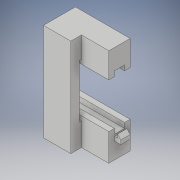
# Autodesk Inventor part: EngineClipTestBlock
Saved by Autodesk Inventor 2018 (Build 220112000, 112)
## iProperties
Created: 2019-08-29
Part Number: EngineClipTestBlock
Material: Generic
Document SubType Name: Modeling
Designer: 871357
Density: 1 g/cm^3
Appearance: Default
Author: 871357
Autodesk Inventor part; units mm, degrees
ref_plane "YZ Plane" through (0, 0, 0) normal (1, 0, 0) x (0, 1, 0)
ref_plane "XZ Plane" through (0, 0, 0) normal (0, 1, 0) x (-1, 0, 0)
sketch "Sketch1" plane through (0, 0, 0) normal (1, 0, 0) x (0, 1, 0)
  line L0 (0, 0) -> (228.6, 0)
  line L1 (228.6, 0) -> (228.6, -424.18)
  line L2 (228.6, -424.18) -> (0, -424.18)
  line L3 (0, -424.18) -> (0, 0)
  point P0 (0, 0)
  dimension "d0" = 424.18
  dimension "d1" = 228.6
  constraints: 8 end point, 2 parallel, 1 coincident, 1 horizontal, 1 perpendicular
  measures "d0" distance of L0.end L1.end
  measures "d1" distance of L0.start L0.end
extrude "Extrusion1" add sketch "Sketch1" along normal blind 165.1
sketch "Sketch2" plane through (165.1, 0, 0) normal (1, 0, 0) x (0, 0, -1)
  line L0 (0, 0) -> (424.18, 0) construction
  line L1 (12.7, 0) -> (411.48, 0)
  line L2 (411.48, 0) -> (411.48, 165.1)
  line L3 (411.48, 165.1) -> (12.7, 165.1)
  line L4 (12.7, 165.1) -> (12.7, 0)
  line L5 (0, 228.6) -> (0, 0) construction
  line L6 (424.18, 0) -> (424.18, 228.6) construction
  dimension "d4" = 398.78
  dimension "d5" = 165.1
  dimension "d6" = 12.7
  dimension "d7" = 12.7
  constraints: 8 end point, 2 parallel, 1 horizontal, 1 perpendicular, 1 point on line
  measures "d4" distance of L3.end L2.end
  measures "d5" distance of L2.end L1.end
  measures "d6" distance between parallel lines of L5 L4
  measures "d7" distance between parallel lines of L6 L2
extrude "Extrusion2" cut sketch "Sketch2" against normal blind 148.59
sketch "Sketch3" plane through (0, 0, 0) normal (0, 0, 1) x (1, 0, 0)
  line L0 (165.1, 228.6) -> (165.1, 0) projected
  line L1 (165.1, 89.535) -> (82.55, 89.535)
  line L2 (69.215, 89.535) -> (69.215, 62.865) construction
  line L3 (82.55, 62.865) -> (165.1, 62.865)
  line L4 (165.1, 62.865) -> (165.1, 89.535)
  line L5 (0, 0) -> (165.1, 0) projected
  arc A0 (82.55, 89.535) -> (82.55, 62.865) centre (82.55, 76.2) ccw
  dimension "d10" = 95.885
  dimension "d11" = 26.67
  dimension "d12" = 62.865
  constraints: 8 end point, 3 tangent, 2 parallel, 2 point on circle, 1 centre point, 1 horizontal, 1 perpendicular, 1 point on line
  measures "d10" distance between parallel lines of L0 L2
  measures "d11" distance of L2.start L2.end
  measures "d12" distance between parallel lines of L5 L3
extrude "Extrusion3" cut sketch "Sketch3" against normal blind 457.2
sketch "Sketch4" plane through (0, 228.6, 0) normal (0, 1, 0) x (1, 0, 0)
  line L0 (165.1, 12.7) -> (165.1, 411.48) construction
  line L1 (165.1, 12.7) -> (16.51, 12.7) construction
  line L2 (16.51, 12.7) -> (16.51, 411.48) construction
  line L3 (165.1, 411.48) -> (16.51, 411.48) construction
  line L4 (0, 424.18) -> (165.1, 424.18) construction
  line L5 (0, 424.18) -> (165.1, 424.18) construction
  circle A0 centre (82.55, 353.06) radius 43.815
  line L6 (0, 0) -> (0, 424.18) construction
  circle A1 centre (82.55, 259.08) radius 43.815
  line L7 (0, 212.09) -> (165.1, 212.09) construction
  line L8 (165.1, 424.18) -> (165.1, 0) construction
  circle A2 centre (82.55, 71.12) radius 43.815
  circle A3 centre (82.55, 165.1) radius 43.815
  dimension "d15" = 87.63
  dimension "d16" = 82.55
  dimension "d17" = 58.42
  dimension "d18" = 87.63
  dimension "d19" = 93.98
  dimension "d20" = 82.55
  constraints: 4 centre point, 4 end point, 2 midpoint, 2 symmetric about line, 1 collinear, 2 other
  measures "d15" diameter of A0
  measures "d16" distance from line of L6 A0.centre
  measures "d17" distance from line of L3 A0.centre
  measures "d18" diameter of A1
  measures "d19" distance of A0.centre A1.centre
  measures "d20" distance from line of L0 A1.centre
extrude "Extrusion4" cut sketch "Sketch4" against normal blind 76.2
sketch "Sketch5" plane through (0, 228.6, 0) normal (0, 1, 0) x (1, 0, 0)
  circle A0 centre (82.55, 165.1) radius 43.815 projected
  circle A1 centre (82.55, 353.06) radius 43.815 projected
  circle A2 centre (82.55, 259.08) radius 43.815 projected
  circle A3 centre (82.55, 71.12) radius 43.815 projected
  line L0 (0, 0) -> (0, 424.18) projected
  line L1 (0, 0) -> (165.1, 0) projected
  line L2 (165.1, 424.18) -> (165.1, 0) projected
  line L3 (0, 424.18) -> (165.1, 424.18) projected
  point P0 (0, 0)
extrude "Extrusion5" add sketch "Sketch5" along normal blind 53.34
sketch "Sketch7" plane through (0, 0, 0) normal (-1, 0, 0) x (0, 0, 1)
  line L0 (0, 0) -> (0, 281.94) projected
  line L1 (-424.18, 281.94) -> (0, 281.94) projected
  line L2 (-424.18, 281.94) -> (-424.18, 0) projected
  line L3 (-424.18, 0) -> (0, 0) projected
  point P0 (0, 0)
extrude "Extrusion6" add sketch "Sketch7" along normal blind 19.05
sketch "Sketch8" plane through (16.51, 0, 0) normal (1, 0, 0) x (0, 0, -1)
  line L0 (411.48, 0) -> (12.7, 0) projected
  line L1 (411.48, 165.1) -> (411.48, 0) projected
  line L2 (12.7, 165.1) -> (411.48, 165.1) projected
  line L3 (12.7, 0) -> (12.7, 165.1) projected
  point P0 (0, 0)
extrude "Extrusion7" cut sketch "Sketch8" against normal blind 19.05
sketch "Sketch12" plane through (165.1, 0, 0) normal (1, 0, 0) x (0, 0, -1)
  line L0 (0, 89.535) -> (12.7, 89.535) construction
  line L1 (3.302, 89.535) -> (9.398, 89.535)
  line L2 (9.398, 89.535) -> (9.398, 92.583)
  line L3 (9.398, 92.583) -> (3.302, 92.583)
  line L4 (3.302, 92.583) -> (3.302, 89.535)
  line L5 (0, 89.535) -> (0, 281.94) construction
  line L6 (12.7, 89.535) -> (12.7, 62.865) construction
  line L7 (0, 89.535) -> (12.7, 89.535) construction
  line L8 (0, 62.865) -> (0, 89.535) construction
  line L9 (0, 62.865) -> (12.7, 62.865) construction
  line L10 (0, 62.865) -> (0, 89.535) construction
  line L11 (0, 76.2) -> (12.7, 76.2) construction
  line L12 (3.302, 62.865) -> (9.398, 62.865)
  line L13 (9.398, 62.865) -> (9.398, 59.817)
  line L14 (9.398, 59.817) -> (3.302, 59.817)
  line L15 (3.302, 59.817) -> (3.302, 62.865)
  point P0 (0, 0)
  dimension "d44" = 6.096
  dimension "d45" = 3.048
  dimension "d46" = 3.302
  constraints: 18 end point, 4 symmetric about line, 2 midpoint, 2 parallel, 1 horizontal, 1 perpendicular, 1 point on line
  measures "d44" distance of L3.end L2.end
  measures "d45" distance of L2.end L1.end
  measures "d46" distance between parallel lines of L5 L4
extrude "Extrusion11" cut sketch "Sketch12" against normal blind 82.55
sketch "Sketch13" plane through (-19.05, 0, 0) normal (0, -1, 0) x (1, 0, 0)
  line L0 (16.51, -12.7) -> (184.15, -12.7) projected
  line L1 (184.15, 0) -> (184.15, -12.7) projected
  line L2 (0, 0) -> (184.15, 0) projected
  line L3 (0, -424.18) -> (0, 0) projected
  line L4 (184.15, -424.18) -> (0, -424.18) projected
  line L5 (184.15, -411.48) -> (184.15, -424.18) projected
  line L6 (184.15, -411.48) -> (16.51, -411.48) projected
  line L7 (16.51, -411.48) -> (16.51, -12.7) projected
  point P0 (19.05, 0)
extrude "Extrusion12" add sketch "Sketch13" along normal blind 5.08
ref_plane "Work Plane1" through (82.55, 89.535, -212.09) normal (0, 0, 1) x (1, 0, 0)
mirror "Mirror1" about plane through (82.55, 89.535, -212.09) normal (0, 0, 1) of "Extrusion11"
sketch "Sketch15" plane through (165.1, 0, 0) normal (1, 0, 0) x (0, 0, -1)
  line L0 (3.302, 59.817) -> (8.89, 59.817)
  line L1 (8.89, 59.817) -> (8.89, 57.912)
  line L2 (8.89, 57.912) -> (3.302, 57.912)
  line L3 (3.302, 57.912) -> (3.302, 59.817)
  line L4 (9.398, 59.817) -> (3.302, 59.817) projected
  point P0 (0, 0)
  dimension "d55" = 5.588
  dimension "d56" = 1.905
  constraints: 8 end point, 2 parallel, 1 horizontal, 1 perpendicular
  measures "d55" distance of L1.end L2.end
  measures "d56" distance of L0.end L1.end
extrude "Extrusion14" add sketch "Sketch15" along normal blind 3.81
sketch "Sketch17" plane through (165.1, 57.912, -3.302) normal (0, 0, 1) x (1, 0, 0)
  line L0 (0, 1.905) -> (3.81, 1.905) projected
  line L1 (3.81, 1.905) -> (0, 1.905)
  line L2 (0, 1.905) -> (0, 0.889)
  line L3 (0, 0.889) -> (3.81, 0.889)
  line L4 (3.81, 0.889) -> (3.81, 1.905)
  point P0 (-165.1, -57.912)
  dimension "d60" = 3.81
  dimension "d61" = 1.016
  constraints: 8 end point, 2 parallel, 1 horizontal, 1 perpendicular
  measures "d60" distance of L3.end L2.end
  measures "d61" distance of L2.end L1.end
extrude "Extrusion15" cut sketch "Sketch17" against normal blind 25.4
sketch "Sketch18" plane through (165.1, 57.912, -3.302) normal (0, 0, 1) x (1, 0, 0)
  line L0 (0, 1.905) -> (-82.55, 1.905) construction
  line L1 (3.81, 0) -> (3.81, 0.889) projected
  line L2 (1.905, 2.9464) -> (3.81, 0.889)
  line L3 (3.81, 0.889) -> (1.905, 0.889)
  line L4 (1.905, 0.889) -> (1.905, 2.9464)
  line L5 (0, 4.953) -> (0, -62.992) projected
  point P0 (-165.1, -57.912)
  dimension "d64" = 1.905
  dimension "d65" = 2.0574
  constraints: 6 end point, 2 perpendicular
  measures "d64" distance between parallel lines of L4 L5
  measures "d65" distance of L3.end L2.start
extrude "Extrusion16" add sketch "Sketch18" against normal blind 5.588
sketch "Sketch19" plane through (165.1, 57.912, -8.89) normal (0, -1, 0) x (1, 0, 0)
  line L0 (0, 0) -> (0, 5.588) projected
  line L1 (0, 0) -> (3.81, 0) projected
  line L2 (3.81, 5.588) -> (3.81, 0) projected
  line L3 (0, 5.588) -> (3.81, 5.588) projected
  point P0 (-165.1, 8.89)
extrude "Extrusion17" add sketch "Sketch19" along normal blind 1.524
mirror "Mirror2" about plane through (82.55, 89.535, -212.09) normal (0, 0, 1) of "Extrusion14", "Extrusion15", "Extrusion16", "Extrusion17"
sketch "Sketch21" plane through (82.55, 89.535, 0) normal (0, 0, 1) x (1, 0, 0)
  line L0 (49.9587, -43.0228) -> (93.9109, -43.0228)
  line L1 (93.9109, -43.0228) -> (93.9109, 15.0648)
  line L2 (93.9109, 15.0648) -> (49.9587, 15.0648)
  line L3 (49.9587, 15.0648) -> (49.9587, -43.0228)
  point P0 (-82.55, -89.535)
  constraints: 8 end point, 2 parallel, 1 horizontal, 1 perpendicular
extrude "Extrusion18" cut sketch "Sketch21" against normal blind 25.4 keep common part
sketch "Sketch22" plane through (132.5087, 104.5998, 0) normal (0, 0, 1) x (1, 0, 0)
  line L0 (0, -58.0876) -> (32.5913, -58.0876) projected
  line L1 (0, 0) -> (16.2957, 0)
  line L2 (16.2957, 0) -> (16.2957, -58.0876)
  line L3 (16.2957, -58.0876) -> (0, -58.0876)
  line L4 (0, -58.0876) -> (0, 0)
  point P0 (-132.5087, -104.5998)
  constraints: 8 end point, 2 parallel, 1 horizontal, 1 midpoint, 1 perpendicular
extrude "Extrusion19" add sketch "Sketch22" along normal blind 6.35
sketch "Sketch23" plane through (148.8043, 62.865, 0) normal (1, 0, 0) x (0, 0, -1)
  line L0 (0, 26.67) -> (0, 41.7348) projected
  line L1 (0, 29.21) -> (-1.27, 29.21)
  line L2 (-1.27, 29.21) -> (-1.27, -2.54)
  line L3 (-1.27, -2.54) -> (0, -2.54)
  line L4 (0, -2.54) -> (0, 29.21)
  line L5 (0, 26.67) -> (3.302, 26.67) projected
  line L6 (3.302, 0) -> (0, 0) projected
  point P0 (0, -62.865)
  dimension "d74" = 1.27
  dimension "d75" = 2.54
  dimension "d76" = 2.54
  constraints: 8 end point, 2 parallel, 1 horizontal, 1 perpendicular, 1 point on line
  measures "d74" distance between parallel lines of L4 L2
  measures "d75" distance between parallel lines of L5 L1
  measures "d76" distance between parallel lines of L6 L3
extrude "Extrusion20" cut sketch "Sketch23" against normal blind 25.4
sketch "Sketch9" plane through (0, 281.94, 0) normal (0, 1, 0) x (1, 0, 0)
  line L0 (146.05, 19.05) -> (146.05, 405.13)
  line L1 (0, 405.13) -> (0, 19.05)
  line L2 (165.1, 424.18) -> (-19.05, 424.18) construction
  line L3 (-19.05, 0) -> (-19.05, 424.18) construction
  line L4 (165.1, 0) -> (165.1, 424.18) construction
  line L5 (165.1, 0) -> (-19.05, 0) construction
  circle A0 centre (82.55, 71.12) radius 43.815 construction
  circle A1 centre (82.55, 259.08) radius 43.815 construction
  circle A2 centre (82.55, 353.06) radius 43.815 construction
  circle A3 centre (82.55, 165.1) radius 43.815 construction
  line L6 (165.1, 0) -> (-19.05, 0) construction
  line L7 (165.1, 0) -> (165.1, 424.18) construction
  line L8 (165.1, 424.18) -> (-19.05, 424.18) construction
  line L9 (-19.05, 0) -> (-19.05, 424.18) construction
  line L10 (146.05, 405.13) -> (117.7739, 405.13)
  line L11 (47.3261, 405.13) -> (0, 405.13)
  arc A4 (47.3261, 405.13) -> (40.7894, 306.07) centre (82.55, 353.06) ccw
  arc A5 (124.3106, 306.07) -> (117.7739, 405.13) centre (82.55, 353.06) ccw
  arc A6 (40.7894, 306.07) -> (40.7894, 212.09) centre (82.55, 259.08) ccw
  arc A7 (124.3106, 212.09) -> (107.2668, 316.8822) centre (82.55, 259.08) ccw
  arc A8 (40.7894, 212.09) -> (40.7894, 118.11) centre (82.55, 165.1) ccw
  arc A9 (124.3106, 118.11) -> (124.3106, 212.09) centre (82.55, 165.1) ccw
  line L12 (0, 19.05) -> (47.3261, 19.05)
  line L13 (117.7739, 19.05) -> (146.05, 19.05)
  arc A10 (40.7894, 118.11) -> (47.3261, 19.05) centre (82.55, 71.12) ccw
  arc A11 (117.7739, 19.05) -> (124.3106, 118.11) centre (82.55, 71.12) ccw
  point P0 (0, 0)
  dimension "d30" = 19.05
  dimension "d31" = 19.05
  constraints: 17 point on circle, 12 end point, 8 centre point, 5 parallel, 4 coincident, 2 horizontal, 2 perpendicular, 2 other
  measures "d30" distance between parallel lines of L3 L1
  measures "d31" distance between parallel lines of L4 L0
sketch "Sketch10" plane through (0, 281.94, -19.05) normal (1, 0, 0) x (0, 0, -1)
  line L0 (405.13, 0) -> (405.13, -281.94) projected
  line L1 (-19.05, 0) -> (405.13, 0) projected
  line L2 (405.13, -101.6) -> (-19.05, -101.6)
  line L3 (-19.05, -101.6) -> (-19.05, 0)
  line L4 (-19.05, 0) -> (405.13, 0)
  line L5 (405.13, 0) -> (405.13, -101.6)
  line L6 (0, 0) -> (386.08, 0) projected
  line L7 (0, 0) -> (0, -101.6) projected
  line L8 (0, -101.6) -> (386.08, -101.6) projected
  line L9 (386.08, 0) -> (386.08, -101.6) projected
  point P0 (-19.05, -281.94)
  dimension "d39" = 0
  constraints: 8 end point, 2 parallel, 1 horizontal, 1 perpendicular, 1 point on line
  measures "d39" distance between parallel lines of L8 L2
sketch "Sketch11" plane through (0, 281.94, 0) normal (0, 1, 0) x (1, 0, 0)
  circle A0 centre (82.55, 71.12) radius 43.815 construction
  line L0 (19.05, 19.05) -> (19.05, 0) projected
  line L1 (19.05, 0) -> (47.3261, 0)
  line L2 (47.3261, 0) -> (47.3261, 19.05)
  line L3 (47.3261, 19.05) -> (19.05, 19.05)
  line L4 (19.05, 19.05) -> (19.05, 0)
  line L5 (165.1, 424.18) -> (19.05, 424.18) projected
  line L6 (47.3261, 405.13) -> (19.05, 405.13)
  line L7 (19.05, 405.13) -> (19.05, 424.18)
  line L8 (19.05, 424.18) -> (47.3261, 424.18)
  line L9 (47.3261, 424.18) -> (47.3261, 405.13)
  point P0 (0, 0)
  constraints: 16 end point, 4 parallel, 2 horizontal, 2 perpendicular
body "Solid1"
